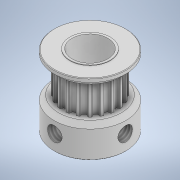
# Autodesk Inventor part: 9mm 20T GT2 Timing Pulley 8mm Bore
Saved by Autodesk Inventor 2020 (Build 240168000, 168)
## iProperties
Created: 2023-06-15
Part Number: 9mm 20T GT2 Timing Pulley 8mm Bore
Material: Generic
Document SubType Name: Modeling
Designer: Ishaan
Density: 1 g/cm^3
Appearance: Default
Author: Ishaan
Autodesk Inventor part; units mm, degrees
sketch "Sketch1" plane through (0, 0, 0) normal (0, 0, 1) x (1, 0, 0)
  line L0 (0, 0) -> (-8, 0)
  line L1 (-8, 0) -> (-8, 7.1)
  line L2 (-8, 7.1) -> (0, 7.1)
  line L3 (0, 7.1) -> (0, 0)
  line L4 (0, 7.1) -> (-6.11, 7.1)
  line L5 (-6.11, 7.1) -> (-6.11, 14.1)
  line L6 (-6.11, 14.1) -> (0, 14.1)
  line L7 (0, 14.1) -> (0, 7.1)
  line L8 (0, 14.1) -> (-8, 14.1)
  line L9 (-8, 14.1) -> (-8, 16)
  line L10 (-8, 16) -> (0, 16)
  line L11 (0, 16) -> (0, 14.1)
  line L12 (0, 16) -> (-4, 16)
  line L13 (-4, 16) -> (-4, 0)
  line L14 (-4, 0) -> (0, 0)
  line L15 (0, 0) -> (0, 16)
  point P0 (-6.11, 7.1)
  dimension "d0" = 8
  dimension "d1" = 4
  dimension "d2" = 16
  dimension "d3" = 7
  dimension "d4" = 7.1
  dimension "d5" = 6.11
  constraints: 32 end point, 8 parallel, 4 horizontal, 4 perpendicular, 1 midpoint, 1 point on line
  measures "d0" distance between parallel lines of L3 L1
  measures "d1" distance between parallel lines of L13 L3
  measures "d2" distance between parallel lines of L0 L10
  measures "d3" distance between parallel lines of L2 L8
  measures "d4" distance between parallel lines of L0 L2
  measures "d5" distance between parallel lines of L7 L5
revolve "Revolution1" add sketch "Sketch1" angle 360 about axis through (0, 0, 0) along (0, 1, 0) contours L0 L1 L2 L13 | L2 L5 L6 L13 | L6 L8 L9 L10 L13
sketch "Sketch2" plane through (0, 16, 0) normal (0, 1, 0) x (1, 0, 0)
  circle A0 centre (0, 0) radius 8 projected
  circle A1 centre (0, 0) radius 4 projected
  circle A2 centre (0, 0) radius 4.5
  dimension "d7" = 0.5
  constraints: 1 centre point
  measures "d7" radial gap between concentric circles of A1 A2
extrude "Extrusion1" cut sketch "Sketch2" against normal blind 0.1 contours A0
ref_plane "Work Plane1" through (0, 8, 0) normal (0, 1, 0) x (1, 0, 0)
mirror "Mirror1" about plane through (0, 8, 0) normal (0, 1, 0) of "Extrusion1"
chamfer "Chamfer2" distance 1 angle 45 2 edges at (8, 14.1, 0) (8, 7.1, 0)
chamfer "Chamfer1" distance 0.125 angle 45 2 edges at (8, 15.9, 0) (8, 0.1, 0)
ref_plane "Work Plane2" through (0, 3.55, 0) normal (0, 1, 0) x (1, 0, 0)
sketch "Sketch3" plane through (0, 0, 0) normal (1, 0, 0) x (0, 1, 0)
  line L0 (3.55, 11.2) -> (3.55, -11.2) projected
  line L1 (-0.61, 0) -> (3.66, 0) projected
  point P0 (0, 0)
  point P1 (3.55, 0)
  constraints: 1 midpoint, 1 point on line
hole "Hole1" at (0, 3.55, 0) direction (1, 0, 0) diameter 3.242 end through all thread size "M4x0.7" class "6H" standard "ANSI Metric M Profile"
ref_plane "Work Plane3" through (0, 0, 0) normal (-0.7071, 0, 0.7071) x (0, -1, 0)
mirror "Mirror2" about plane through (0, 0, 0) normal (-0.7071, 0, 0.7071) of "Hole1"
sketch "Sketch5" plane through (0, 14.1, 0) normal (0, -1, 0) x (1, 0, 0)
  circle A0 centre (0, 0) radius 6.11 projected
  circle A1 centre (0, 0) radius 4 projected
  circle A2 centre (0, 0) radius 6.11 construction
  circle A3 centre (0, 0) radius 6.11 construction
  arc A4 (-0.7227, -6.0671) -> (0.7227, -6.0671) centre (0, 0) ccw
  arc A5 (0.555, -5.9175) -> (0.7227, -6.0671) centre (0.705, -5.9182) ccw
  arc A6 (-0.7227, -6.0671) -> (-0.555, -5.9175) centre (-0.705, -5.9182) ccw
  arc A7 (0.555, -5.9175) -> (-0.555, -5.9175) centre (0, -5.915) ccw
  circle A8 centre (0, 0) radius 7 projected
  point P0 (0.7227, -6.0671)
  dimension "d22" = 12.22
  dimension "d23" = 0.15
  dimension "d24" = 0.555
  dimension "d25" = 0.75
  constraints: 8 point on circle, 5 centre point, 5 tangent, 1 coincident, 1 concentric, 1 equal radius, 1 vertical alignment
  measures "d22" diameter of A3
  measures "d23" radius of A5
  measures "d24" radius of A7
extrude "Extrusion2" cut sketch "Sketch5" along normal up to surface (7 mm away) contours A6 A7 A5 A0 picked at (-0.0224, -5.8582)
pattern_circular "Circular Pattern1" count 20 over 360 about axis through (0, 8, 0) along (0, 1, 0) of "Extrusion2"
body "Solid1"
